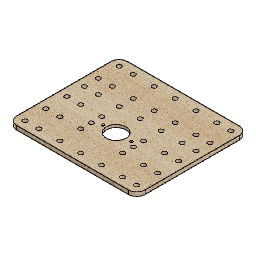
model (Autodesk Fusion 360 design; units mm, degrees)
Autodesk Fusion 360 part; units mm, degrees
sketch "bench" plane through (0, 0, 0) normal (0, 0, 1) x (1, 0, 0)
  line L0 (0, 0) -> (608, 0)
  line L1 (608, 0) -> (608, 448)
  line L2 (608, 448) -> (0, 448)
  line L3 (0, 448) -> (0, 0)
  circle A0 centre (112, 112) radius 10
  circle A1 centre (208, 112) radius 10
  circle A2 centre (304, 112) radius 10
  circle A3 centre (400, 112) radius 10
  circle A4 centre (496, 112) radius 10
  circle A5 centre (112, 208) radius 10
  circle A6 centre (208, 208) radius 10
  circle A7 centre (304, 208) radius 10
  circle A8 centre (400, 208) radius 10
  circle A9 centre (496, 208) radius 10
  circle A10 centre (112, 304) radius 10
  circle A11 centre (208, 304) radius 10
  circle A12 centre (304, 304) radius 10
  circle A13 centre (400, 304) radius 10
  circle A14 centre (496, 304) radius 10
  circle A15 centre (112, 400) radius 10
  circle A16 centre (208, 400) radius 10
  circle A17 centre (304, 400) radius 10
  circle A18 centre (400, 400) radius 10
  circle A19 centre (496, 400) radius 10
  circle A20 centre (560, 400) radius 10
  circle A21 centre (560, 304) radius 10
  circle A22 centre (560, 208) radius 10
  circle A23 centre (560, 112) radius 10
  circle A24 centre (48, 400) radius 10
  circle A25 centre (48, 304) radius 10
  circle A26 centre (48, 208) radius 10
  circle A27 centre (48, 112) radius 10
  circle A28 centre (48, 48) radius 10
  circle A29 centre (112, 48) radius 10
  circle A30 centre (208, 48) radius 10
  circle A31 centre (304, 48) radius 10
  circle A32 centre (400, 48) radius 10
  circle A33 centre (560, 48) radius 10
  circle A34 centre (496, 48) radius 10
  line L4 (48, 48) -> (0, 48) construction
  line L5 (48, 48) -> (48, 0) construction
  line L6 (560, 48) -> (608, 48) construction
  line L7 (48, 400) -> (48, 448) construction
  dimension "d1" = 20
  dimension "d4" = 96
  dimension "d5" = 96
  dimension "d8" = 64
  dimension "d9" = 0
  dimension "d12" = -64
  dimension "d13" = 0
  dimension "d16" = 0
  dimension "d17" = -64
  dimension "d18" = 48
  constraint horizontal L0
  constraint vertical L1
  constraint horizontal L2
  constraint vertical L3
  constraint coincident L0.start L3.end
  constraint coincident A28.centre L4.start
  constraint coincident L3 L4.end
  constraint coincident L0 L5.end
  constraint horizontal L4
  constraint vertical L5
  constraint equal L4 L5
  constraint coincident A33.centre L6.start
  constraint coincident L1 L6.end
  constraint horizontal L6
  constraint equal L4 L6
  constraint coincident A24.centre L7.start
  constraint coincident L2 L7.end
  constraint vertical L7
  constraint equal L5 L7
  measures "d1" diameter of A0
  measures "d18" distance of L0.start L4.end
sketch "table" plane through (0, 0, 0) normal (0, 0, 1) x (1, 0, 0)
  line L0 (10, 246) -> (598, 246)
  line L1 (598, 246) -> (598, -262)
  line L2 (598, -262) -> (10, -262)
  line L3 (10, -262) -> (10, 246)
  line L4 (304, -62.1314) -> (304, -262) construction
  line L5 (304, 246) -> (304, 400) construction
  line L6 (248, -5) -> (360, -5)
  arc A0 (248, -5) -> (360, -5) centre (304, -62.1314) ccw
  line L7 (48, 208) -> (10, 208) construction
  line L8 (48, 208) -> (48, 246) construction
  arc A1 (48, 246) -> (10, 208) centre (48, 208) ccw
  arc A2 (598, 208) -> (560, 246) centre (560, 208) ccw
  arc A3 (560, -262) -> (598, -224) centre (560, -224) ccw
  arc A4 (10, -224) -> (48, -262) centre (48, -224) ccw
  circle A5 centre (48, 208) radius 10
  circle A6 centre (48, 112) radius 10
  circle A7 centre (112, 112) radius 10
  circle A8 centre (112, 208) radius 10
  circle A9 centre (208, 208) radius 10
  circle A10 centre (208, 112) radius 10
  circle A11 centre (48, 48) radius 10
  circle A12 centre (112, 48) radius 10
  circle A13 centre (208, 48) radius 10
  circle A14 centre (304, 112) radius 10
  circle A15 centre (304, 208) radius 10
  circle A16 centre (304, 48) radius 10
  circle A17 centre (400, 48) radius 10
  circle A18 centre (400, 112) radius 10
  circle A19 centre (400, 208) radius 10
  circle A20 centre (496, 208) radius 10
  circle A21 centre (496, 112) radius 10
  circle A22 centre (496, 48) radius 10
  circle A23 centre (560, 112) radius 10
  circle A24 centre (560, 208) radius 10
  circle A25 centre (560, 48) radius 10
  circle A26 centre (48, 16) radius 10
  circle A27 centre (112, 16) radius 10
  circle A28 centre (208, 16) radius 10
  circle A29 centre (304, 16) radius 10
  circle A30 centre (400, 16) radius 10
  circle A31 centre (496, 16) radius 10
  circle A32 centre (560, 16) radius 10
  circle A33 centre (48, -80) radius 10
  circle A34 centre (112, -80) radius 10
  circle A35 centre (208, -80) radius 10
  circle A36 centre (304, -80) radius 10
  circle A37 centre (400, -80) radius 10
  circle A38 centre (496, -80) radius 10
  circle A39 centre (560, -80) radius 10
  circle A40 centre (48, -176) radius 10
  circle A41 centre (112, -176) radius 10
  circle A42 centre (208, -176) radius 10
  circle A43 centre (304, -176) radius 10
  circle A44 centre (400, -176) radius 10
  circle A45 centre (496, -176) radius 10
  circle A46 centre (560, -176) radius 10
  circle A47 centre (48, -32) radius 10
  circle A48 centre (112, -32) radius 10
  circle A49 centre (208, -32) radius 10
  circle A50 centre (304, -32) radius 10
  circle A51 centre (400, -32) radius 10
  circle A52 centre (496, -32) radius 10
  circle A53 centre (560, -32) radius 10
  circle A54 centre (48, -128) radius 10
  circle A55 centre (112, -128) radius 10
  circle A56 centre (208, -128) radius 10
  circle A57 centre (304, -128) radius 10
  circle A58 centre (400, -128) radius 10
  circle A59 centre (496, -128) radius 10
  circle A60 centre (560, -128) radius 10
  circle A61 centre (48, -224) radius 10
  circle A62 centre (112, -224) radius 10
  circle A63 centre (208, -224) radius 10
  circle A64 centre (304, -224) radius 10
  circle A65 centre (400, -224) radius 10
  circle A66 centre (496, -224) radius 10
  circle A67 centre (560, -224) radius 10
  circle A68 centre (304, -62.1314) radius 45
  line L9 (224, -62.1314) -> (384, -62.1314) construction
  circle A69 centre (374, -62.1314) radius 3.175
  circle A70 centre (374, -62.1314) radius 6.5
  circle A71 centre (244, -62.1314) radius 6.5
  circle A72 centre (244, -62.1314) radius 3.175
  point P0 (304, -62.1314)
  point P1 (304, 400)
  point P2 (496, 208)
  point P3 (48, 208)
  point P4 (48, 112)
  dimension "d23" = 508
  dimension "d24" = 588
  dimension "d26" = 160
  dimension "d29" = 102
  dimension "d30" = 112
  dimension "d31" = 199.8686
  dimension "d34" = 0
  dimension "d35" = -96
  dimension "d40" = 5
  dimension "d43" = 0
  dimension "d44" = 48
  dimension "d47" = 0
  dimension "d48" = -48
  dimension "d54" = 90
  dimension "d55" = 6.35
  dimension "d56" = 13
  dimension "d57" = 10
  dimension "d58" = 130
  constraint horizontal L0
  constraint vertical L1
  constraint horizontal L2
  constraint vertical L3
  constraint coincident P0 L4.start
  constraint midpoint L2 L4.end
  constraint vertical L4
  constraint midpoint L0 L5.start
  constraint coincident P1 L5.end
  constraint vertical L5
  constraint horizontal L6
  constraint coincident P3 L7.start
  constraint coincident L3 L7.end
  constraint coincident L0 L8.end
  constraint horizontal L7
  constraint vertical L8
  constraint equal L7 L8
  constraint tangent L0 A1
  constraint tangent L3 A1
  constraint tangent L0 A2
  constraint coincident L1 A2.start
  constraint coincident L0 A2.end
  constraint tangent L1 A3
  constraint coincident L1 A3.end
  constraint coincident L2 A3.start
  constraint tangent L2 A4
  constraint coincident L2 A4.end
  constraint coincident L3 A4.start
  constraint tangent L3 A4
  constraint tangent L2 A3
  constraint tangent L1 A2
  constraint equal A1 A2
  constraint equal A1 A4
  constraint equal A1 A3
  constraint concentric A0 A68
  constraint coincident A0 L9.start
  constraint coincident A0 L9.end
  constraint horizontal L9
  constraint coincident P0 L9
  constraint coincident L9 A69.centre
  constraint concentric A69 A70
  constraint coincident L9 A71.centre
  constraint concentric A71 A72
  constraint equal A69 A72
  constraint equal A70 A71
  measures "d23" distance of L0.start L2.end
  measures "d24" distance of L0.start L0.end
  measures "d26" diameter of A0
  measures "d29" distance of L1 P2
  measures "d30" distance of L6.start L6.end
  measures "d31" distance of P0 L4.end
  measures "d40" vertical distance of L6.start origin
  measures "d54" diameter of A68
  measures "d55" diameter of A69
  measures "d56" diameter of A70
  measures "d57" distance of L9.end A69.centre
  measures "d58" distance of A69.centre A71.centre
extrude "Extrude1" add sketch "table" against normal blind 18 contours L0 L1 L2 L3 A1 A2 A3 A4 | L6 A0 | A5 | A6 | A7 | A8 | A9 | A10 | A11 | A12 | A13 | A14 | A15 | A16 | A17 | A18 | A19 | A20 | A21 | A22 | A23 | A24 | A25 | A26 | A27 | A28 | A29 | A30 | A31 | A32 | A33 | A34 | A35 | A36 | A37 | A38 | A39 | A40 | A41 | A42 | A43 | A44 | A45 | A46 | A47 | A48 | A49 | A50 | A51 | A52 | A53 | A54 | A55 | A56 | A57 | A58 | A59 | A60 | A61 | A62 | A63 | A64 | A65 | A66 | A67 | A68 | A69 | A70 | A71 | A72
extrude "Extrude2" cut sketch "bench" sketch "table" against normal blind 25 contours A0 | A1 | A2 | A3 | A4 | A5 | A6 | A7 | A8 | A9 | A22 | A23 | A27 | A28 | A29 | A30 | A31 | A32 | A33 | A34 of sketch 2 contours A5 | A35 | A36 | A37 | A47 | A48 | A49 | A50 | A51 | A52 | A53 | A54 | A55 | A56 | A58 | A59 | A60 | A61 | A62 | A63 | A64 | A65 | A66 | A67 | A68 | A69 | A72
extrude "Extrude3" cut sketch "table" against normal blind 6.5 contours A70 | A71
extrude "Extrude4" cut sketch "table" along normal blind 6 from surface at -18 contours L6 A0 | A57 | A70 | A71
equation "maxA = 608 mm - margin - 5 mm"
equation "maxB = 523 mm - margin"
equation "d23 = maxB"
equation "d24 = maxA"
equation "margin = 15 mm"
